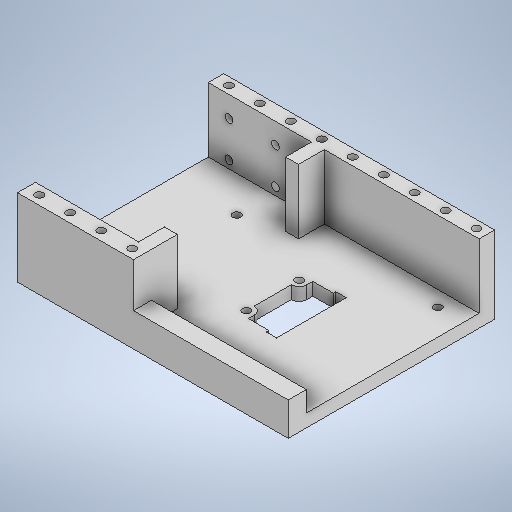
# Autodesk Inventor part: sensor_zig
Saved by Autodesk Inventor 2025 (Build 290162010, 162A)
## iProperties
Created: 2024-10-24
Part Number: sensor_zig
Material: Generic
Document SubType Name: Modeling
Designer: fist5
Density: 1 g/cm^3
Appearance: Default
Author: fist5
Autodesk Inventor part; units mm, degrees
ref_plane "YZ Plane" through (0, 0, 0) normal (1, 0, 0) x (0, 1, 0)
ref_plane "XZ Plane" through (0, 0, 0) normal (0, 1, 0) x (-1, 0, 0)
ref_plane "XY Plane" through (0, 0, 0) normal (0, 0, 1) x (1, 0, 0)
sketch "Sketch1" plane through (0, 0, 0) normal (0, 1, 0) x (-1, 0, 0)
  line L0 (0, 0) -> (105, 0)
  line L1 (105, 0) -> (105, -80)
  line L2 (105, -80) -> (0, -80)
  line L3 (0, -80) -> (0, 0)
  dimension "d0" = 105
  dimension "d1" = 80
  constraints: 8 end point, 2 parallel, 1 horizontal, 1 perpendicular
  measures "d0" distance between parallel lines of L1 L3
  measures "d1" distance between parallel lines of L2 L0
extrude "Extrusion1" add sketch "Sketch1" along normal blind 5
sketch "Sketch2" plane through (0, 5, 0) normal (0, 1, 0) x (1, 0, 0)
  line L0 (0, 0) -> (0, 80) projected
  line L1 (-105, 80) -> (-105, 0) projected
  line L2 (0, 74) -> (-105, 74)
  line L3 (-105, 74) -> (-105, 7)
  line L4 (-105, 7) -> (0, 7)
  line L5 (0, 7) -> (0, 74)
  line L6 (-105, 0) -> (0, 0) projected
  line L7 (0, 80) -> (-105, 80) projected
  line L8 (-60, 7) -> (-60, 0)
  line L9 (-60, 7) -> (-65, 7)
  line L10 (-65, 7) -> (-65, 74)
  line L11 (-65, 74) -> (-60, 74)
  line L12 (-60, 74) -> (-60, 7)
  line L13 (-60, 64) -> (-65, 64)
  line L14 (-65, 64) -> (-65, 17)
  line L15 (-65, 17) -> (-60, 17)
  line L16 (-60, 17) -> (-60, 64)
  line L17 (0, 80) -> (-105, 80) projected
  line L18 (-105, 80) -> (-105, 0) projected
  line L19 (-105, 0) -> (0, 0) projected
  line L20 (0, 0) -> (0, 80) projected
  point P0 (-62.5, 74)
  point P1 (-62.5, 64)
  point P2 (-62.5, 7)
  point P3 (-62.5, 17)
  dimension "d4" = 7
  dimension "d5" = 6
  dimension "d7" = 45
  dimension "d8" = 5
  dimension "d9" = 10
  dimension "d10" = 10
  constraints: 26 end point, 7 point on line, 6 parallel, 4 midpoint, 4 perpendicular, 3 horizontal
  measures "d4" distance between parallel lines of L6 L4
  measures "d5" distance between parallel lines of L7 L2
  measures "d7" distance between parallel lines of L1 L8
  measures "d8" distance between parallel lines of L10 L12
  measures "d9" distance of point (-62.5, 74) point (-62.5, 64)
  measures "d10" distance of point (-62.5, 7) point (-62.5, 17)
extrude "Extrusion2" add sketch "Sketch2" along normal blind 25 contours L6 L1 L4 L8 | L2 L1 L7 L0 | L4 L10 L15 L12 | L12 L13 L10 L2
sketch "Sketch3" plane through (0, 30, 0) normal (0, 1, 0) x (1, 0, 0)
  line L0 (-100, 3.5) -> (-5, 3.5)
  line L1 (-5, 3.5) -> (-5, 77)
  line L2 (-5, 77) -> (-100, 77)
  line L3 (-100, 77) -> (-100, 3.5)
  line L4 (0, 80) -> (-105, 80) projected
  line L5 (-105, 0) -> (-60, 0) projected
  line L6 (-105, 74) -> (-105, 7) projected
  line L7 (0, 0) -> (0, 74) projected
  circle A0 centre (-100, 3.5) radius 1.5
  circle A1 centre (-100, 77) radius 1.5
  dimension "d13" = 3
  dimension "d14" = 3.5
  dimension "d15" = 5
  dimension "d16" = 5
  dimension "d17" = 3
  dimension "d20" = 3
  constraints: 8 end point, 2 centre point, 2 coincident, 2 parallel, 1 horizontal, 1 perpendicular
  measures "d13" distance between parallel lines of L4 L2
  measures "d14" distance between parallel lines of L5 L0
  measures "d15" distance between parallel lines of L3 L6
  measures "d16" distance between parallel lines of L7 L1
  measures "d17" diameter of A0
  measures "d20" diameter of A1
extrude "Extrusion3" cut sketch "Sketch3" against normal blind 10 contours L3 A0 L0 | L0 A0 L3
extrude "Extrusion4" cut sketch "Sketch3" against normal blind 10 contours A1 L2 L3 | L3 L2 A1
pattern_linear "Rectangular Pattern2" count 4 spacing 12 along (1, 0, 0) of "Extrusion3"
pattern_linear "Rectangular Pattern3" count 9 spacing 12 along (1, 0, 0) of "Extrusion4"
sketch "Sketch4" plane through (0, 0, 0) normal (0, -1, 0) x (1, 0, 0)
  line L0 (-10, -12) -> (-80, -12)
  line L1 (-80, -12) -> (-80, -68)
  line L2 (-80, -68) -> (-10, -68)
  line L3 (-10, -68) -> (-10, -12)
  line L4 (0, -80) -> (-105, -80) projected
  line L5 (0, 0) -> (0, -80) projected
  line L6 (-80, -60) -> (-10, -68)
  line L7 (-10, -12) -> (-80, -20)
  circle A0 centre (-10, -12) radius 1.5
  circle A1 centre (-10, -68) radius 1.5
  circle A2 centre (-80, -20) radius 1.5
  circle A3 centre (-80, -60) radius 1.5
  point P0 (-80, -40)
  point P1 (-45, -68)
  point P2 (-11.5, -12)
  point P3 (-11.4903, -12.1703)
  dimension "d32" = 70
  dimension "d33" = 40
  dimension "d34" = 45
  dimension "d35" = 56
  dimension "d36" = 40
  dimension "d37" = 20
  dimension "d38" = 3
  dimension "d39" = 3
  dimension "d40" = 3
  dimension "d41" = 3
  constraints: 12 end point, 4 centre point, 4 coincident, 2 midpoint, 2 parallel, 2 point on line, 1 horizontal, 1 perpendicular
  measures "d32" distance between parallel lines of L1 L3
  measures "d33" distance from line of L4 point (-80, -40)
  measures "d34" distance from line of L5 point (-45, -68)
  measures "d35" distance between parallel lines of L2 L0
  measures "d36" distance of L6.start L7.end
  measures "d37" distance of L6.start point (-80, -40)
  measures "d38" diameter of A0
  measures "d39" diameter of A1
  measures "d40" diameter of A3
  measures "d41" diameter of A2
extrude "Extrusion5" cut sketch "Sketch4" against normal up to next contours L7 A0 L0 | L0 A0 L3 | L3 A0 L7 | A1 L2 L3 | L3 L6 A1 | A2 L1 L7 | L7 L1 A2 | L1 A2 | L2 A1 L6 | A3 L1 L6 | L6 L1 A3 | L1 A3
sketch "Sketch5" plane through (0, 5, 0) normal (0, 1, 0) x (1, 0, 0)
  line L0 (-105, 0) -> (0, 0) projected
  line L1 (0, 0) -> (-61.099, 0)
  line L2 (-61.099, 0) -> (-61.099, 7)
  line L3 (-61.099, 7) -> (0, 7)
  line L4 (0, 7) -> (0, 0)
  point P0 (-105, 7)
  constraints: 8 end point, 2 parallel, 1 horizontal, 1 horizontal alignment, 1 perpendicular
extrude "Extrusion6" add sketch "Sketch5" along normal blind 7.9
sketch "Sketch6" plane through (0, 0, -80) normal (0, 0, -1) x (-1, 0, 0)
  line L0 (97, 22) -> (79, 22)
  line L1 (79, 22) -> (79, 8)
  line L2 (79, 8) -> (97, 8)
  line L3 (97, 8) -> (97, 22)
  line L4 (0, 0) -> (105, 0) projected
  line L5 (0, 0) -> (0, 30) projected
  circle A0 centre (97, 8) radius 1.5
  circle A1 centre (97, 22) radius 1.5
  circle A2 centre (79, 22) radius 1.5
  circle A3 centre (79, 8) radius 1.5
  line L6 (105, 0) -> (105, 30) projected
  point P0 (79, 15)
  point P1 (105, 15)
  dimension "d46" = 15
  dimension "d47" = 14
  dimension "d48" = 18
  dimension "d50" = 3
  dimension "d51" = 3
  dimension "d52" = 3
  dimension "d53" = 3
  dimension "d56" = 8
  constraints: 8 end point, 4 centre point, 4 coincident, 2 midpoint, 2 parallel, 1 horizontal, 1 perpendicular
  measures "d46" distance from line of L4 point (79, 15)
  measures "d47" distance between parallel lines of L2 L0
  measures "d48" distance between parallel lines of L1 L3
  measures "d50" diameter of A0
  measures "d51" diameter of A1
  measures "d52" diameter of A2
  measures "d53" diameter of A3
  measures "d56" distance from line of point (105, 15) L3
extrude "Extrusion7" cut sketch "Sketch6" against normal up to surface (6 mm away) contours A2 L1 L0 | L0 L1 A2 | A1 L3 L0 | L0 L3 A1 | A3 L2 L1 | L1 L2 A3 | A0 L2 L3 | L3 L2 A0
sketch "Sketch7" plane through (0, 0, 0) normal (0, -1, 0) x (1, 0, 0)
  line L0 (-32, -27.5) -> (-48, -27.5)
  line L1 (-48, -27.5) -> (-48, -52.5)
  line L2 (-48, -52.5) -> (-32, -52.5)
  line L3 (-32, -52.5) -> (-32, -27.5)
  line L4 (0, 0) -> (0, -80) projected
  line L5 (-105, 0) -> (0, 0) projected
  line L6 (-46, -27.5) -> (-46, -52.5)
  line L7 (-44, -27.5) -> (-44, -52.5)
  circle A0 centre (-46, -29.75) radius 1.5
  circle A1 centre (-46, -50.25) radius 1.5
  circle A2 centre (-46, -50.25) radius 3.0104
  circle A3 centre (-46, -29.75) radius 3.0104
  line L8 (-42.9896, -50.25) -> (-42.9896, -52.5)
  line L9 (-42.9896, -29.75) -> (-42.9896, -27.5)
  point P0 (-40, -52.5)
  point P1 (-32, -40)
  point P2 (-46, -40)
  point P3 (-48, -40)
  point P4 (-46, -32.7604)
  point P5 (-46, -47.2396)
  dimension "d57" = 40
  dimension "d58" = 40
  dimension "d59" = 25
  dimension "d60" = 16
  dimension "d62" = 2
  dimension "d63" = 4
  dimension "d64" = 3
  dimension "d65" = 2.25
  dimension "d66" = 2.25
  dimension "d67" = 3
  constraints: 16 end point, 8 point on line, 4 centre point, 4 midpoint, 4 point on circle, 3 perpendicular, 2 coincident, 2 parallel, 1 horizontal, 1 horizontal alignment, 1 tangent, 1 vertical
  measures "d57" distance from line of L4 point (-40, -52.5)
  measures "d58" distance from line of L5 point (-32, -40)
  measures "d59" distance between parallel lines of L2 L0
  measures "d60" distance between parallel lines of L1 L3
  measures "d62" distance between parallel lines of L1 L6
  measures "d63" distance between parallel lines of L1 L7
  measures "d64" diameter of A0
  measures "d65" distance from line of L0 A0.centre
  measures "d66" distance from line of L2 A1.centre
  measures "d67" diameter of A1
extrude "Extrusion8" cut sketch "Sketch7" against normal up to surface (5 mm away) contours L3 L2 L8 A2 L7 A3 L9 L0 | L7 A2 L6 A3 | A0 L6 | L6 A0 | A1 L6 | L6 A1
sketch "Sketch8" plane through (0, 0, 0) normal (0, -1, 0) x (1, 0, 0)
  line L0 (-31, -53.5) -> (-35, -53.5)
  line L1 (-35, -53.5) -> (-35, -26.5)
  line L2 (-35, -26.5) -> (-31, -26.5)
  line L3 (-31, -26.5) -> (-31, -53.5)
  line L4 (-32, -52.5) -> (-42.9896, -52.5) projected
  line L5 (-42.9896, -27.5) -> (-32, -27.5) projected
  line L6 (-32, -27.5) -> (-32, -52.5) projected
  point P0 (0, 0)
  point P1 (-33, -53.5)
  dimension "d70" = 1
  dimension "d71" = 1
  dimension "d72" = 4
  dimension "d73" = 1
  constraints: 8 end point, 2 parallel, 1 horizontal, 1 midpoint, 1 perpendicular
  measures "d70" distance from line of point (-33, -53.5) L4
  measures "d71" distance between parallel lines of L5 L2
  measures "d72" distance between parallel lines of L3 L1
  measures "d73" distance between parallel lines of L6 L3
extrude "Extrusion9" cut sketch "Sketch8" against normal up to surface (5 mm away)
equation "\"d54\" = d52"
body "Solid1"
